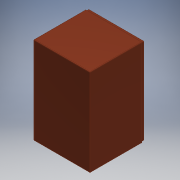
# Autodesk Inventor part: NP12-12FR Battery
Saved by Autodesk Inventor 2018 (Build 220112000, 112)
## iProperties
Created: 2017-10-31
Part Number: NP12-12FR Battery
Material: Copper
Document SubType Name: Modeling
Designer: P136265
Density: 8.94 g/cm^3
Appearance: Copper - Satin
Author: P136265
Autodesk Inventor part; units mm, degrees
ref_plane "YZ Plane" through (0, 0, 0) normal (1, 0, 0) x (0, 1, 0)
ref_plane "XZ Plane" through (0, 0, 0) normal (0, 1, 0) x (-1, 0, 0)
ref_plane "XY Plane" through (0, 0, 0) normal (0, 0, 1) x (1, 0, 0)
sketch "Sketch1" plane through (0, 0, 0) normal (0, 1, 0) x (-1, 0, 0)
  line L0 (-48.5, 75) -> (48.5, 75)
  line L1 (48.5, 75) -> (48.5, -75)
  line L2 (48.5, -75) -> (-48.5, -75)
  line L3 (-48.5, -75) -> (-48.5, 75)
  line L4 (-48.5, 75) -> (48.5, -75) construction
  line L5 (48.5, 75) -> (-48.5, -75) construction
  point P0 (0, 0)
  dimension "d0" = 97
  dimension "d1" = 150
  constraints: 12 end point, 2 midpoint, 2 parallel, 1 horizontal, 1 perpendicular
  measures "d0" distance of L1.end L2.end
  measures "d1" distance of L0.end L1.end
extrude "Extrusion1" add sketch "Sketch1" along normal blind 94
sketch "Sketch2" plane through (0, 94, 0) normal (0, 1, 0) x (1, 0, 0)
  line L0 (-48.5, -75) -> (48.5, -75) construction
  line L1 (48.5, -75) -> (48.5, 75) construction
  line L2 (48.5, 75) -> (-48.5, 75) construction
  line L3 (-48.5, 75) -> (-48.5, -75) construction
  line L4 (-47.5, -74) -> (47.5, -74)
  line L5 (47.5, -74) -> (47.5, 74)
  line L6 (47.5, 74) -> (-47.5, 74)
  line L7 (-47.5, 74) -> (-47.5, -74)
  line L8 (-48.5, 75) -> (-48.5, -75) projected
  line L9 (-48.5, -75) -> (48.5, -75)
  line L10 (48.5, -75) -> (48.5, 75)
  line L11 (48.5, 75) -> (-48.5, 75)
  line L12 (-48.5, 75) -> (-48.5, -75)
  point P0 (0, 0)
  dimension "d4" = 1
  constraints: 16 end point, 2 parallel, 1 horizontal, 1 perpendicular, 3 other
  measures "d4" distance between parallel lines of L3 L7
extrude "Extrusion2" cut sketch "Sketch2" against normal blind 5
fillet "Fillet1" radius 1 16 edges at (48.5, 44.5, -75) (48.5, 44.5, 75) (-48.5, 44.5, -75) (-48.5, 44.5, 75) (0, 0, 75) (-48.5, 0, 0) (0, 0, -75) (48.5, 0, 0) (47.5, 91.5, -74) (47.5, 94, 0) (0, 94, -74) (47.5, 91.5, 74) (-47.5, 91.5, 74) (0, 94, 74) (-47.5, 94, 0) (-47.5, 91.5, -74)
sketch "Sketch3" plane through (0, 94, 0) normal (0, 1, 0) x (1, 0, 0)
  line L0 (47.5, -73) -> (47.5, 73) construction
  line L1 (-46.5, -74) -> (46.5, -74) construction
  line L2 (-47.5, 73) -> (-47.5, -73) construction
  line L3 (-42.5, -63) -> (-36.5, -63)
  line L4 (-36.5, -63) -> (-36.5, -62)
  line L5 (-36.5, -62) -> (-42.5, -62)
  line L6 (-42.5, -62) -> (-42.5, -63)
  line L7 (-42.5, -63) -> (-36.5, -62) construction
  line L8 (-36.5, -63) -> (-42.5, -62) construction
  line L9 (36.5, -63) -> (42.5, -63)
  line L10 (42.5, -63) -> (42.5, -62)
  line L11 (42.5, -62) -> (36.5, -62)
  line L12 (36.5, -62) -> (36.5, -63)
  line L13 (36.5, -63) -> (42.5, -62) construction
  line L14 (42.5, -63) -> (36.5, -62) construction
  point P0 (0, 0)
  point P1 (-39.5, -62.5)
  point P2 (39.5, -62.5)
  dimension "d12" = 6
  dimension "d13" = 1
  dimension "d14" = 6
  dimension "d15" = 1
  dimension "d16" = 11
  dimension "d17" = 5
  dimension "d18" = 5
  dimension "d19" = 11
  constraints: 24 end point, 4 midpoint, 4 parallel, 2 horizontal, 2 perpendicular
  measures "d12" distance of L5.end L4.end
  measures "d13" distance of L4.end L3.end
  measures "d14" distance of L11.end L10.end
  measures "d15" distance of L10.end L9.end
  measures "d16" distance between parallel lines of L1 L9
  measures "d17" distance between parallel lines of L0 L10
  measures "d18" distance between parallel lines of L2 L6
  measures "d19" distance between parallel lines of L1 L3
extrude "Extrusion3" add sketch "Sketch3" along normal blind 3
sketch "Sketch4" plane through (42.5, 94, 62) normal (0, 0, -1) x (-1, 0, 0)
  line L0 (-0.25, 2) -> (6.25, 2)
  line L1 (6.25, 2) -> (6.25, 3)
  line L2 (6.25, 3) -> (-0.25, 3)
  line L3 (-0.25, 3) -> (-0.25, 2)
  line L4 (-0.25, 2) -> (6.25, 3) construction
  line L5 (6.25, 2) -> (-0.25, 3) construction
  line L6 (0, 3) -> (6, 3) construction
  line L7 (78.75, 2) -> (85.25, 2)
  line L8 (85.25, 2) -> (85.25, 3)
  line L9 (85.25, 3) -> (78.75, 3)
  line L10 (78.75, 3) -> (78.75, 2)
  line L11 (78.75, 2) -> (85.25, 3) construction
  line L12 (85.25, 2) -> (78.75, 3) construction
  line L13 (79, 3) -> (85, 3) construction
  point P0 (42.5, -94)
  point P1 (3, 2.5)
  point P2 (3, 3)
  point P3 (82, 2.5)
  point P4 (82, 3)
  dimension "d22" = 6.5
  dimension "d23" = 1
  dimension "d24" = 6.5
  dimension "d25" = 1
  constraints: 24 end point, 8 midpoint, 4 parallel, 2 horizontal, 2 perpendicular
  measures "d22" distance of L2.end L1.end
  measures "d23" distance of L1.end L0.end
  measures "d24" distance of L9.end L8.end
  measures "d25" distance of L8.end L7.end
extrude "Extrusion4" add sketch "Sketch4" along normal blind 10
fillet "Fillet2" radius 0.25 28 edges at (42.75, 96.5, 52) (36.25, 96.5, 52) (42.75, 96.5, 62) (36.25, 96.5, 62) (-36.25, 96.5, 52) (-36.25, 96.5, 62) (-42.75, 96.5, 52) (-42.75, 96.5, 62) (-42.75, 97, 57) (-42.75, 96, 57) (-39.5, 97, 52) (-39.5, 96, 52) (-36.25, 96, 57) (-36.25, 97, 57) (-36.5, 95, 62) (-36.5, 95.5, 63) (-42.5, 95, 62) (-42.5, 95.5, 63) (42.75, 97, 57) (42.75, 96, 57) (42.5, 95, 62) (42.5, 95.5, 63) (39.5, 97, 52) (39.5, 96, 52) (36.25, 97, 57) (36.25, 96, 57) (36.5, 95, 62) (36.5, 95.5, 63)
fillet "Fillet2" radius 1 2 edges at (39.5, 97, 63) (-39.5, 97, 63)
sketch "Sketch5" plane through (0, 94, 0) normal (0, 1, 0) x (1, 0, 0)
  line L0 (-46.5, -74) -> (46.5, -74) construction
  line L1 (-47.5, 73) -> (-47.5, -73) construction
  line L2 (47.5, -73) -> (47.5, 73) construction
  line L3 (25.5, -70) -> (25.5, -64) construction
  line L4 (-25.5, -70) -> (-25.5, -64) construction
  line L5 (-28.5, -67) -> (-22.5, -67) construction
  line L6 (-25.85, -69.9795) -> (-25.85, -67.35)
  line L7 (-25.85, -66.65) -> (-25.85, -64.0205)
  line L8 (-25.15, -69.9795) -> (-25.15, -67.35)
  line L9 (-25.15, -66.65) -> (-25.15, -64.0205)
  line L10 (-28.4795, -66.65) -> (-25.85, -66.65)
  line L11 (-25.15, -66.65) -> (-22.5205, -66.65)
  line L12 (-28.4795, -67.35) -> (-25.85, -67.35)
  line L13 (-25.15, -67.35) -> (-22.5205, -67.35)
  arc A0 (-25.85, -64.0205) -> (-28.4795, -66.65) centre (-25.5, -67) ccw
  arc A1 (-22.5205, -66.65) -> (-25.15, -64.0205) centre (-25.5, -67) ccw
  arc A2 (-28.4795, -67.35) -> (-25.85, -69.9795) centre (-25.5, -67) ccw
  arc A3 (-25.15, -69.9795) -> (-22.5205, -67.35) centre (-25.5, -67) ccw
  line L14 (25.15, -69.9795) -> (25.15, -64.0205)
  line L15 (25.85, -69.9795) -> (25.85, -64.0205)
  arc A4 (25.15, -64.0205) -> (25.15, -69.9795) centre (25.5, -67) ccw
  arc A5 (25.85, -69.9795) -> (25.85, -64.0205) centre (25.5, -67) ccw
  point P0 (0, 0)
  dimension "d32" = 7
  dimension "d33" = 22
  dimension "d34" = 7
  dimension "d35" = 22
  dimension "d40" = 3
  dimension "d41" = 3
  dimension "d42" = 3
  dimension "d43" = 3
  dimension "d44" = 0.7
  dimension "d45" = 0.7
  dimension "d46" = 0.7
  dimension "d47" = 0.7
  dimension "d48" = 72.65
  dimension "d49" = 72.65
  dimension "d50" = 73
  dimension "d51" = 22
  dimension "d52" = 7.35
  dimension "d53" = 7
  dimension "d54" = 7.35
  dimension "d55" = 70
  dimension "d56" = 10
  dimension "d57" = 4
  dimension "d58" = 76
  dimension "d59" = 0.35
  dimension "d60" = 0.35
  dimension "d61" = 3
  dimension "d62" = 3
  dimension "d63" = 10
  dimension "d64" = 4
  constraints: 26 end point, 12 point on circle, 11 parallel, 6 centre point, 1 horizontal, 1 vertical
  measures "d32" distance from line of L0 A4.centre
  measures "d33" distance from line of L2 A4.centre
  measures "d34" distance from line of L0 A0.centre
  measures "d35" distance from line of L1 A0.centre
  measures "d40" radius of A0
  measures "d41" radius of A1
  measures "d42" radius of A2
  measures "d43" radius of A3
  measures "d44" distance between parallel lines of L12 L10
  measures "d45" distance between parallel lines of L13 L11
  measures "d46" distance between parallel lines of L7 L9
  measures "d47" distance between parallel lines of L6 L8
  measures "d48" distance between parallel lines of L2 L9
  measures "d49" distance between parallel lines of L2 L8
  measures "d50" distance between parallel lines of L2 L4
  measures "d51" distance between parallel lines of L3 L2
  measures "d52" distance between parallel lines of L11 L0
  measures "d53" distance between parallel lines of L5 L0
  measures "d54" distance between parallel lines of L10 L0
  measures "d55" distance from line of L5.end L2
  measures "d56" distance from line of L4.end L0
  measures "d57" distance from line of L4.start L0
  measures "d58" distance from line of L5.start L2
  measures "d59" distance between parallel lines of L3 L14
  measures "d60" distance between parallel lines of L3 L15
  measures "d61" radius of A4
  measures "d62" radius of A5
  measures "d63" distance from line of L3.end L0
  measures "d64" distance from line of L3.start L0
extrude "Extrusion5" cut sketch "Sketch5" against normal blind 0.2
body "Solid1"
